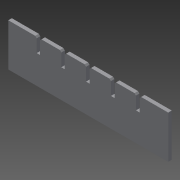
# Autodesk Inventor part: SlotRuler
Saved by Autodesk Inventor 2015 (Build 190159000, 159)
## iProperties
Created: 2015-02-15
Part Number: SlotRuler
Material: Generic
Document SubType Name: Modeling
Designer: Iain
Density: 1 g/cm^3
Appearance: Default
Author: Iain
Autodesk Inventor part; units mm, degrees
ref_plane "YZ Plane" through (0, 0, 0) normal (1, 0, 0) x (0, 1, 0)
ref_plane "XZ Plane" through (0, 0, 0) normal (0, 1, 0) x (-1, 0, 0)
ref_plane "XY Plane" through (0, 0, 0) normal (0, 0, 1) x (1, 0, 0)
sketch "Sketch1" plane through (0, 0, 0) normal (0, 1, 0) x (-1, 0, 0)
  line L0 (75, -15) -> (-75, -15)
  line L1 (-75, -15) -> (-75, 15)
  line L2 (-75, 15) -> (75, 15)
  line L3 (75, 15) -> (75, -15)
  point P0 (0, 0)
  point P1 (0, -15)
  point P2 (75, 0)
  point P3 (0, 15)
  dimension "d0" = 150
  dimension "d1" = 30
  constraints: 8 end point, 3 midpoint, 2 parallel, 1 horizontal, 1 horizontal alignment, 1 perpendicular, 1 vertical alignment
  measures "d0" distance of L1.end L2.end
  measures "d1" distance of L2.end L0.start
extrude "Extrusion1" add sketch "Sketch1" along normal blind 2.5
sketch "Sketch3" plane through (0, 2.5, 0) normal (0, 1, 0) x (1, 0, 0)
  line L0 (-75, 15) -> (-75, -15) projected
  line L1 (-75, -15) -> (75, -15) projected
  line L2 (-55, -15) -> (-52.7, -15)
  line L3 (-52.7, -15) -> (-52.7, -5)
  line L4 (-52.7, -5) -> (-55, -5)
  line L5 (-55, -5) -> (-55, -15)
  point P0 (0, 0)
  point P1 (-53.85, -15)
  point P2 (0, -15)
  dimension "d4" = 2.3
  dimension "d5" = 10
  dimension "d6" = 20
  constraints: 8 end point, 2 midpoint, 2 parallel, 1 horizontal, 1 horizontal alignment, 1 perpendicular
  measures "d4" distance of L3.end L4.end
  measures "d5" distance of L4.end L2.start
  measures "d6" distance from line of L0 L4.end
extrude "-0.2" cut sketch "Sketch3" along normal through all both and the other way through all
sketch "Sketch4" plane through (0, 2.5, 0) normal (0, 1, 0) x (1, 0, 0)
  line L0 (-75, -15) -> (-55, -15) projected
  line L1 (-37.7, -5) -> (-35.3, -5)
  line L2 (-35.3, -5) -> (-35.3, -15)
  line L3 (-35.3, -15) -> (-37.7, -15)
  line L4 (-37.7, -15) -> (-37.7, -5)
  point P0 (-52.7, -15)
  point P1 (0, 0)
  point P2 (-36.5, -15)
  point P3 (-65, -15)
  dimension "d9" = 10
  dimension "d10" = 2.4
  dimension "d11" = 15
  constraints: 8 end point, 2 midpoint, 2 parallel, 1 horizontal, 1 horizontal alignment, 1 perpendicular
  measures "d9" distance of L3.end L1.start
  measures "d10" distance of L1.start L1.end
  measures "d11" distance of point (-52.7, -15) L3.end
extrude "-0.1" cut sketch "Sketch4" against normal through all
sketch "Sketch5" plane through (0, 2.5, 0) normal (0, 1, 0) x (1, 0, 0)
  line L0 (-75, -15) -> (-55, -15) projected
  line L1 (-20.3, -5) -> (-17.8, -5)
  line L2 (-17.8, -5) -> (-17.8, -15)
  line L3 (-17.8, -15) -> (-20.3, -15)
  line L4 (-20.3, -15) -> (-20.3, -5)
  point P0 (-35.3, -5)
  point P1 (0, 0)
  point P2 (-19.05, -15)
  point P3 (-65, -15)
  dimension "d15" = 10
  dimension "d16" = 2.5
  dimension "d17" = 15
  constraints: 8 end point, 2 midpoint, 2 parallel, 1 horizontal, 1 horizontal alignment, 1 perpendicular
  measures "d15" distance of L1.end L2.end
  measures "d16" distance of L1.start L1.end
  measures "d17" distance of point (-35.3, -5) L1.start
extrude "0.0" cut sketch "Sketch5" against normal through all
sketch "Sketch6" plane through (0, 2.5, 0) normal (0, 1, 0) x (1, 0, 0)
  line L0 (-75, -15) -> (-55, -15) projected
  line L1 (-2.8, -15) -> (-0.2, -15)
  line L2 (-0.2, -15) -> (-0.2, -5)
  line L3 (-0.2, -5) -> (-2.8, -5)
  line L4 (-2.8, -5) -> (-2.8, -15)
  point P0 (-17.8, -5)
  point P1 (0, 0)
  point P2 (-1.5, -15)
  point P3 (-65, -15)
  dimension "d20" = 10
  dimension "d21" = 2.6
  dimension "d22" = 15
  constraints: 8 end point, 2 midpoint, 2 parallel, 1 horizontal, 1 horizontal alignment, 1 perpendicular
  measures "d20" distance of L1.end L2.end
  measures "d21" distance of L2.end L3.end
  measures "d22" distance of point (-17.8, -5) L3.end
extrude "+0.1" cut sketch "Sketch6" against normal through all
sketch "Sketch7" plane through (0, 2.5, 0) normal (0, 1, 0) x (1, 0, 0)
  line L0 (-75, -15) -> (-55, -15) projected
  line L1 (14.8, -15) -> (17.5, -15)
  line L2 (17.5, -15) -> (17.5, -5)
  line L3 (17.5, -5) -> (14.8, -5)
  line L4 (14.8, -5) -> (14.8, -15)
  point P0 (-0.2, -5)
  point P1 (0, 0)
  point P2 (16.15, -15)
  point P3 (-65, -15)
  dimension "d25" = 10
  dimension "d26" = 2.7
  dimension "d27" = 15
  constraints: 8 end point, 2 midpoint, 2 parallel, 1 horizontal, 1 horizontal alignment, 1 perpendicular
  measures "d25" distance of L1.end L2.end
  measures "d26" distance of L2.end L3.end
  measures "d27" distance of point (-0.2, -5) L3.end
extrude "+0.2" cut sketch "Sketch7" against normal through all
sketch "Sketch8" plane through (0, 2.5, 0) normal (0, 1, 0) x (1, 0, 0)
  line L0 (75, 15) -> (-75, 15) projected
  line L1 (-75, 15) -> (-75, -15) projected
  line L2 (-75, -15) -> (-55, -15) projected
  line L3 (-75, 15) -> (37.5, 15)
  line L4 (37.5, 15) -> (37.5, -15)
  line L5 (37.5, -15) -> (-75, -15)
  line L6 (-75, -15) -> (-75, 15)
  point P0 (17.5, -5)
  point P1 (0, 0)
  point P2 (-18.75, -15)
  point P3 (-65, -15)
  point P4 (-18.75, 15)
  point P5 (0, 15)
  point P6 (-75, 0)
  point P7 (-75, 0)
  dimension "d30" = 20
  constraints: 8 end point, 6 midpoint, 2 horizontal alignment, 2 parallel, 1 coincident, 1 horizontal, 1 perpendicular
  measures "d30" distance from line of L4 point (17.5, -5)
extrude "Extrusion7" cut sketch "Sketch8" against normal through all keep common part
chamfer "Chamfer1" distance 1 angle 45 10 edges at (-55, 1.25, 15) (-52.7, 1.25, 15) (-37.7, 1.25, 15) (-35.3, 1.25, 15) (-20.3, 1.25, 15) (-17.8, 1.25, 15) (-2.8, 1.25, 15) (-0.2, 1.25, 15) (14.8, 1.25, 15) (17.5, 1.25, 15)
equation "\"d2\" = CardThickness"
equation "\"d12\" = CardThickness"
equation "\"d16\" = CardThickness"
equation "\"d18\" = CardThickness"
equation "\"d23\" = CardThickness"
equation "\"d28\" = CardThickness"
equation "\"d31\" = CardThickness"
equation "\"CardThickness\" = 2.5"
body "Solid1"
